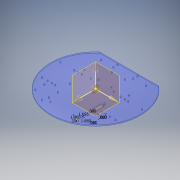
# Autodesk Inventor part: TopPlate
Saved by Autodesk Inventor 2019 (Build 230136000, 136)
## iProperties
Created: 2020-02-28
Part Number: TopPlate
Material: Generic
Document SubType Name: Modeling
Designer: james
Mass: 617.778 g
Surface Area: 2655.15 cm^2
Volume: 617.778 cm^3
Density: 1 g/cm^3
Appearance: Clear - Blue
Author: james
Autodesk Inventor part; units mm, degrees
ref_plane "YZ Plane" through (0, 0, 0) normal (1, 0, 0) x (0, 1, 0)
ref_plane "XZ Plane" through (0, 0, 0) normal (0, 1, 0) x (-1, 0, 0)
ref_plane "XY Plane" through (0, 0, 0) normal (0, 0, 1) x (1, 0, 0)
sketch "Sketch1" plane through (0, 0, 0) normal (0, 1, 0) x (-1, 0, 0)
  circle A0 centre (0, 0) radius 203.2
  dimension "d0" = 406.4
  constraints: 1 centre point, 1 coincident
  measures "d0" diameter of A0
extrude "Extrusion1" add sketch "Sketch1" along normal blind 4.7625
sketch "Sketch6" plane through (0, 0, 0) normal (0, -1, 0) x (1, 0, 0)
  point P0 (0, 0)
  point P1 (52.197, 152.4)
  point P2 (-52.197, 152.4)
  dimension "d48" = 0
  dimension "d49" = 104.394
  dimension "d50" = 52.197
  dimension "d51" = 152.4
  measures "d48" vertical distance of point (-52.197, 152.4) point (52.197, 152.4)
  measures "d49" distance of point (-52.197, 152.4) point (52.197, 152.4)
  measures "d50" horizontal distance of point (0, 0) point (52.197, 152.4)
  measures "d51" vertical distance of point (0, 0) point (-52.197, 152.4)
hole "Hole3" at (52.197, 0, 152.4) at (-52.197, 0, 152.4) direction (0, 1, 0) diameter 3.81 depth 25.4 tip angle 118
sketch "Sketch8" plane through (0, 4.7625, 0) normal (0, 1, 0) x (1, 0, 0)
  line L0 (-249.9736, 258.2829) -> (238.9858, 258.2829)
  line L1 (238.9858, 258.2829) -> (238.9858, 152.4)
  line L2 (238.9858, 152.4) -> (-249.9736, 152.4)
  line L3 (-249.9736, 152.4) -> (-249.9736, 258.2829)
  point P0 (0, 0)
  dimension "d80" = 152.4
  constraints: 8 end point, 2 parallel, 1 horizontal, 1 perpendicular
  measures "d80" distance from line of point (0, 0) L2
extrude "Extrusion4" cut sketch "Sketch8" against normal blind 100.0125
sketch "Sketch14" plane through (0, 4.7625, 0) normal (0, 1, 0) x (1, 0, 0)
  circle A0 centre (52.197, -152.4) radius 1.905 projected
  circle A1 centre (-52.197, -152.4) radius 1.905 projected
  point P0 (0, 0)
  point P1 (-52.197, 29.87)
  point P2 (52.197, 29.87)
  dimension "d138" = 0
  dimension "d139" = 182.27
  dimension "d140" = 182.27
  dimension "d141" = 0
  measures "d138" horizontal distance of A1.centre point (-52.197, 29.87)
  measures "d139" distance of A1.centre point (-52.197, 29.87)
  measures "d140" distance of A0.centre point (52.197, 29.87)
  measures "d141" horizontal distance of A0.centre point (52.197, 29.87)
hole "Hole7" at (-52.197, 4.7625, -29.87) at (52.197, 4.7625, -29.87) direction (0, -1, 0) diameter 5.1054 depth 25.4 tip angle 118 clearance for "Hex Machine Screw" size "#10" standard "Ansi Unified Screw Threads"
sketch "Sketch15" plane through (0, 4.7625, 0) normal (0, 1, 0) x (1, 0, 0)
  circle A0 centre (-52.197, -152.4) radius 1.905 projected
  point P0 (0, 0)
  point P1 (-78.74, -165.1)
  point P2 (-78.74, -38.1)
  point P3 (78.74, -165.1)
  point P4 (78.74, -38.1)
  dimension "d149" = 0
  dimension "d150" = 0
  dimension "d151" = 0
  dimension "d152" = 0
  dimension "d153" = 127
  dimension "d155" = 157.48
  dimension "d156" = 78.74
  dimension "d270" = 12.7
  measures "d149" vertical distance of point (78.74, -38.1) point (-78.74, -38.1)
  measures "d150" vertical distance of point (78.74, -165.1) point (-78.74, -165.1)
  measures "d151" horizontal distance of point (78.74, -165.1) point (78.74, -38.1)
  measures "d152" horizontal distance of point (-78.74, -165.1) point (-78.74, -38.1)
  measures "d153" distance of point (-78.74, -38.1) point (-78.74, -165.1)
  measures "d155" distance of point (78.74, -165.1) point (-78.74, -165.1)
  measures "d156" horizontal distance of point (0, 0) point (-78.74, -38.1)
  measures "d270" vertical distance of point (-78.74, -165.1) A0.centre
hole "Hole8" at (-78.74, 4.7625, 165.1) at (-78.74, 4.7625, 38.1) at (78.74, 4.7625, 165.1) at (78.74, 4.7625, 38.1) direction (0, -1, 0) diameter 5.1054 depth 25.4 tip angle 118 clearance for "Flat Head Machine Screw (82)" size "#10" standard "Ansi Unified Screw Threads"
sketch "Sketch16" plane through (0, 4.7625, 0) normal (0, 1, 0) x (1, 0, 0)
  circle A0 centre (78.74, -165.1) radius 2.5527 projected
  point P0 (0, 0)
  point P1 (81.28, -96.647)
  point P2 (129.032, -96.647)
  point P3 (81.28, -139.7)
  point P4 (129.032, -139.7)
  dimension "d164" = 0
  dimension "d165" = 0
  dimension "d166" = 0
  dimension "d167" = 0
  dimension "d170" = 47.752
  dimension "d171" = 43.053
  dimension "d271" = 2.54
  dimension "d272" = 25.4
  measures "d164" horizontal distance of point (129.032, -139.7) point (129.032, -96.647)
  measures "d165" horizontal distance of point (81.28, -139.7) point (81.28, -96.647)
  measures "d166" vertical distance of point (129.032, -96.647) point (81.28, -96.647)
  measures "d167" vertical distance of point (81.28, -139.7) point (129.032, -139.7)
  measures "d170" distance of point (129.032, -139.7) point (81.28, -139.7)
  measures "d171" distance of point (81.28, -139.7) point (81.28, -96.647)
  measures "d271" horizontal distance of A0.centre point (81.28, -139.7)
  measures "d272" vertical distance of A0.centre point (81.28, -139.7)
hole "Hole9" at (81.28, 4.7625, 96.647) at (129.032, 4.7625, 96.647) at (81.28, 4.7625, 139.7) at (129.032, 4.7625, 139.7) direction (0, -1, 0) diameter 5.1054 depth 25.4 tip angle 118 clearance for "Flat Head Machine Screw (82)" size "#10" standard "Ansi Unified Screw Threads"
sketch "Sketch17" plane through (0, 4.7625, 0) normal (0, 1, 0) x (1, 0, 0)
  circle A0 centre (-52.197, 29.87) radius 2.5527 projected
  point P0 (0, 0)
  point P1 (-29.5275, 102.9204)
  point P2 (-29.5275, 42.57)
  point P3 (29.5275, 42.57)
  point P4 (29.5275, 102.9204)
  dimension "d179" = 0
  dimension "d180" = 0
  dimension "d181" = 0
  dimension "d182" = 0
  dimension "d183" = 59.055
  dimension "d184" = 29.5275
  dimension "d185" = 12.7
  dimension "d186" = 60.3504
  measures "d179" vertical distance of point (29.528, 102.92) point (-29.528, 102.92)
  measures "d180" vertical distance of point (-29.528, 42.57) point (29.528, 42.57)
  measures "d181" horizontal distance of point (29.528, 102.92) point (29.528, 42.57)
  measures "d182" horizontal distance of point (-29.528, 102.92) point (-29.528, 42.57)
  measures "d183" distance of point (29.528, 42.57) point (-29.528, 42.57)
  measures "d184" horizontal distance of point (0, 0) point (-29.528, 42.57)
  measures "d185" vertical distance of A0.centre point (-29.528, 42.57)
  measures "d186" distance of point (-29.528, 42.57) point (-29.528, 102.92)
hole "Hole10" at (-29.5275, 4.7625, -102.9204) at (-29.5275, 4.7625, -42.57) at (29.5275, 4.7625, -42.57) at (29.5275, 4.7625, -102.9204) direction (0, -1, 0) diameter 5.1054 depth 25.4 tip angle 118 clearance for "Flat Head Machine Screw (82)" size "#10" standard "Ansi Unified Screw Threads"
sketch "Sketch18" plane through (0, 4.7625, 0) normal (0, 1, 0) x (1, 0, 0)
  line L0 (134.4042, 152.4) -> (-134.4042, 152.4) projected
  point P0 (0, 0)
  point P1 (-45.085, 144.78)
  point P2 (45.085, 144.78)
  point P3 (45.085, 125.73)
  point P4 (-45.085, 125.73)
  dimension "d194" = 90.17
  dimension "d195" = 0
  dimension "d196" = 19.05
  dimension "d197" = 0
  dimension "d198" = 0
  dimension "d199" = 0
  dimension "d200" = 7.62
  dimension "d201" = 45.085
  measures "d194" distance of point (45.085, 144.78) point (-45.085, 144.78)
  measures "d195" vertical distance of point (45.085, 144.78) point (-45.085, 144.78)
  measures "d196" distance of point (45.085, 125.73) point (45.085, 144.78)
  measures "d197" horizontal distance of point (45.085, 125.73) point (45.085, 144.78)
  measures "d198" vertical distance of point (-45.085, 125.73) point (45.085, 125.73)
  measures "d199" horizontal distance of point (-45.085, 125.73) point (-45.085, 144.78)
  measures "d200" distance from line of L0 point (-45.085, 144.78)
  measures "d201" horizontal distance of point (-45.085, 125.73) point (0, 0)
hole "Hole11" at (-45.085, 4.7625, -144.78) at (45.085, 4.7625, -144.78) at (45.085, 4.7625, -125.73) at (-45.085, 4.7625, -125.73) direction (0, -1, 0) diameter 5.1054 depth 25.4 tip angle 118 clearance for "Flat Head Machine Screw (82)" size "#10" standard "Ansi Unified Screw Threads"
sketch "Sketch19" plane through (0, 4.7625, 0) normal (0, 1, 0) x (1, 0, 0)
  point P0 (0, 0)
  point P1 (-106.68, -76.2)
  point P2 (-121.92, -76.2)
  point P3 (106.68, -76.2)
  point P4 (121.92, -76.2)
  dimension "d209" = 0
  dimension "d210" = 76.2
  dimension "d211" = 76.2
  dimension "d212" = 0
  dimension "d213" = 15.24
  dimension "d214" = 15.24
  dimension "d215" = 106.68
  dimension "d216" = 106.68
  measures "d209" vertical distance of point (106.68, -76.2) point (121.92, -76.2)
  measures "d210" vertical distance of point (0, 0) point (106.68, -76.2)
  measures "d211" vertical distance of point (-106.68, -76.2) point (0, 0)
  measures "d212" vertical distance of point (-121.92, -76.2) point (-106.68, -76.2)
  measures "d213" distance of point (-106.68, -76.2) point (-121.92, -76.2)
  measures "d214" distance of point (121.92, -76.2) point (106.68, -76.2)
  measures "d215" horizontal distance of point (0, 0) point (-106.68, -76.2)
  measures "d216" horizontal distance of point (0, 0) point (106.68, -76.2)
hole "Hole12" at (-106.68, 4.7625, 76.2) at (-121.92, 4.7625, 76.2) at (106.68, 4.7625, 76.2) at (121.92, 4.7625, 76.2) direction (0, -1, 0) diameter 5.1054 depth 25.4 tip angle 118 clearance for "Flat Head Machine Screw (82)" size "#10" standard "Ansi Unified Screw Threads"
sketch "Sketch20" plane through (0, 4.7625, 0) normal (0, 1, 0) x (1, 0, 0)
  circle A0 centre (-121.92, -76.2) radius 2.5527 projected
  circle A1 centre (-106.68, -76.2) radius 2.5527 projected
  circle A2 centre (106.68, -76.2) radius 2.5527 projected
  circle A3 centre (121.92, -76.2) radius 2.5527 projected
  circle A4 centre (121.92, -76.2) radius 2.5527 projected
  point P0 (0, 0)
  point P1 (-121.92, 25.4)
  point P2 (-106.68, 25.4)
  point P3 (121.92, 25.4)
  point P4 (106.68, 25.4)
  dimension "d224" = 0
  dimension "d225" = 0
  dimension "d226" = 0
  dimension "d227" = 0
  dimension "d228" = 0
  dimension "d229" = 0
  dimension "d230" = 0
  dimension "d231" = 101.6
  measures "d224" vertical distance of point (106.68, 25.4) point (121.92, 25.4)
  measures "d225" horizontal distance of A3.centre point (121.92, 25.4)
  measures "d226" horizontal distance of A2.centre point (106.68, 25.4)
  measures "d227" horizontal distance of A1.centre point (-106.68, 25.4)
  measures "d228" horizontal distance of A0.centre point (-121.92, 25.4)
  measures "d229" vertical distance of point (-106.68, 25.4) point (-121.92, 25.4)
  measures "d230" vertical distance of point (106.68, 25.4) point (-121.92, 25.4)
  measures "d231" distance of point (121.92, 25.4) A3.centre
hole "Hole13" at (-121.92, 4.7625, -25.4) at (-106.68, 4.7625, -25.4) at (121.92, 4.7625, -25.4) at (106.68, 4.7625, -25.4) direction (0, -1, 0) diameter 5.1054 depth 25.4 tip angle 118 clearance for "Flat Head Machine Screw (82)" size "#10" standard "Ansi Unified Screw Threads"
sketch "Sketch21" plane through (0, 4.7625, 0) normal (0, 1, 0) x (1, 0, 0)
  circle A0 centre (121.92, 25.4) radius 2.5527 projected
  circle A1 centre (106.68, 25.4) radius 2.5527 projected
  circle A2 centre (-106.68, 25.4) radius 2.5527 projected
  circle A3 centre (-121.92, 25.4) radius 2.5527 projected
  point P0 (0, 0)
  point P1 (-87.63, 25.4)
  point P2 (-185.42, 25.4)
  point P3 (87.63, 25.4)
  point P4 (185.42, 25.4)
  dimension "d239" = 0
  dimension "d240" = 0
  dimension "d241" = 0
  dimension "d242" = 0
  dimension "d243" = 19.05
  dimension "d244" = 63.5
  dimension "d245" = 63.5
  dimension "d246" = 19.05
  measures "d239" vertical distance of point (185.42, 25.4) A0.centre
  measures "d240" vertical distance of A1.centre point (87.63, 25.4)
  measures "d241" vertical distance of A2.centre point (-87.63, 25.4)
  measures "d242" vertical distance of point (-185.42, 25.4) A3.centre
  measures "d243" distance of A2.centre point (-87.63, 25.4)
  measures "d244" distance of point (-185.42, 25.4) A3.centre
  measures "d245" distance of A0.centre point (185.42, 25.4)
  measures "d246" distance of point (87.63, 25.4) A1.centre
hole "Hole14" at (-87.63, 4.7625, -25.4) at (-185.42, 4.7625, -25.4) at (87.63, 4.7625, -25.4) at (185.42, 4.7625, -25.4) direction (0, -1, 0) diameter 5.1054 depth 25.4 tip angle 118 clearance for "Flat Head Machine Screw (82)" size "#10" standard "Ansi Unified Screw Threads"
sketch "Sketch22" plane through (0, 4.7625, 0) normal (0, 1, 0) x (1, 0, 0)
  circle A0 centre (-121.92, -76.2) radius 2.5527 projected
  circle A1 centre (-106.68, -76.2) radius 2.5527 projected
  circle A2 centre (106.68, -76.2) radius 2.5527 projected
  circle A3 centre (121.92, -76.2) radius 2.5527 projected
  point P0 (0, 0)
  point P1 (-140.97, -76.2)
  point P2 (-166.37, -76.2)
  point P3 (140.97, -76.2)
  point P4 (166.37, -76.2)
  dimension "d254" = 0
  dimension "d255" = 0
  dimension "d256" = 19.05
  dimension "d257" = 25.4
  dimension "d258" = 0
  dimension "d259" = 0
  dimension "d260" = 25.4
  dimension "d261" = 19.05
  measures "d254" vertical distance of point (-140.97, -76.2) A0.centre
  measures "d255" vertical distance of A0.centre point (-166.37, -76.2)
  measures "d256" distance of point (-140.97, -76.2) A0.centre
  measures "d257" distance of point (-166.37, -76.2) point (-140.97, -76.2)
  measures "d258" vertical distance of point (140.97, -76.2) A3.centre
  measures "d259" vertical distance of A3.centre point (166.37, -76.2)
  measures "d260" distance of point (140.97, -76.2) point (166.37, -76.2)
  measures "d261" distance of A3.centre point (140.97, -76.2)
hole "Hole15" at (-140.97, 4.7625, 76.2) at (-166.37, 4.7625, 76.2) at (140.97, 4.7625, 76.2) at (166.37, 4.7625, 76.2) direction (0, -1, 0) diameter 5.1054 depth 25.4 tip angle 118 clearance for "Flat Head Machine Screw (82)" size "#10" standard "Ansi Unified Screw Threads"
sketch "Sketch23" plane through (0, 4.7625, 0) normal (0, 1, 0) x (1, 0, 0)
  line L0 (75.8881, -46.5788) -> (84.511, -46.5788)
  line L1 (87.686, -49.7538) -> (87.686, -83.9555)
  line L2 (84.511, -87.1305) -> (75.8881, -87.1305)
  line L3 (72.7131, -83.9555) -> (72.7131, -49.7538)
  arc A0 (87.686, -49.7538) -> (84.511, -46.5788) centre (84.511, -49.7538) ccw
  arc A1 (84.511, -87.1305) -> (87.686, -83.9555) centre (84.511, -83.9555) ccw
  arc A2 (72.7131, -83.9555) -> (75.8881, -87.1305) centre (75.8881, -83.9555) ccw
  arc A3 (75.8881, -46.5788) -> (72.7131, -49.7538) centre (75.8881, -49.7538) ccw
  point P0 (0, 0)
  dimension "d273" = 3.175
  constraints: 8 end point, 8 point on circle, 8 tangent, 4 centre point, 3 equal radius, 2 parallel, 1 horizontal, 1 perpendicular
  measures "d273" radius of A0
extrude "Extrusion8" cut sketch "Sketch23" against normal blind 25.4
sketch "Sketch24" plane through (0, 4.7625, 0) normal (0, 1, 0) x (1, 0, 0)
  circle A0 centre (-78.74, -165.1) radius 2.5527 projected
  point P0 (0, 0)
  point P1 (-133.35, -99.06)
  point P2 (-72.39, -99.06)
  point P3 (-133.35, -139.7)
  point P4 (-72.39, -139.7)
  dimension "d276" = 40.64
  dimension "d277" = 60.96
  dimension "d278" = 0
  dimension "d279" = 0
  dimension "d280" = 0
  dimension "d281" = 0
  dimension "d289" = 25.4
  dimension "d290" = 6.35
  measures "d276" distance of point (-72.39, -139.7) point (-72.39, -99.06)
  measures "d277" distance of point (-133.35, -99.06) point (-72.39, -99.06)
  measures "d278" vertical distance of point (-133.35, -99.06) point (-72.39, -99.06)
  measures "d279" vertical distance of point (-72.39, -139.7) point (-133.35, -139.7)
  measures "d280" horizontal distance of point (-133.35, -99.06) point (-133.35, -139.7)
  measures "d281" horizontal distance of point (-72.39, -139.7) point (-72.39, -99.06)
  measures "d289" vertical distance of point (-72.39, -139.7) A0.centre
  measures "d290" horizontal distance of A0.centre point (-72.39, -139.7)
hole "Hole16" at (-133.35, 4.7625, 99.06) at (-72.39, 4.7625, 99.06) at (-72.39, 4.7625, 139.7) at (-133.35, 4.7625, 139.7) direction (0, -1, 0) diameter 5.1054 depth 25.4 tip angle 118 clearance for "Flat Head Machine Screw (82)" size "#10" standard "Ansi Unified Screw Threads"
sketch "Sketch25" plane through (0, 0, 0) normal (0, -1, 0) x (1, 0, 0)
  point P0 (0, 0)
  point P1 (-101.6, -50.8)
  point P2 (-101.6, -127)
  point P3 (101.6, -127)
  point P4 (101.6, -50.8)
  dimension "d291" = 0
  dimension "d292" = 0
  dimension "d293" = 0
  dimension "d294" = 0
  dimension "d295" = 101.6
  dimension "d296" = 101.6
  dimension "d297" = 76.2
  dimension "d298" = 50.8
  measures "d291" vertical distance of point (101.6, -50.8) point (-101.6, -50.8)
  measures "d292" vertical distance of point (101.6, -127) point (-101.6, -127)
  measures "d293" horizontal distance of point (101.6, -50.8) point (101.6, -127)
  measures "d294" horizontal distance of point (-101.6, -50.8) point (-101.6, -127)
  measures "d295" horizontal distance of point (-101.6, -50.8) point (0, 0)
  measures "d296" horizontal distance of point (101.6, -50.8) point (0, 0)
  measures "d297" distance of point (101.6, -127) point (101.6, -50.8)
  measures "d298" vertical distance of point (0, 0) point (-101.6, -50.8)
hole "Hole17" at (-101.6, 0, -50.8) at (-101.6, 0, -127) at (101.6, 0, -127) at (101.6, 0, -50.8) direction (0, 1, 0) diameter 5.1054 depth 25.4 tip angle 118 clearance for "Flat Head Machine Screw (82)" size "#10" standard "Ansi Unified Screw Threads"
body "Solid1"
